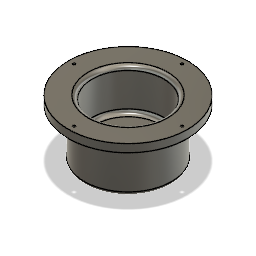
distance sensing base v1 (Autodesk Fusion 360 design; units mm, degrees)
Autodesk Fusion 360 part; units mm, degrees
note: some values were not read from the file. Set by a fixed rule: which sketch regions a step uses.
sketch "Sketch1" plane through (0, 0, 0) normal (0, 0, 1) x (1, 0, 0)
  line L0 (0, 0) -> (0, -69.4878)
  line L1 (15, -30) -> (25, -50)
  line L2 (15, -30) -> (40, -30)
  line L3 (25, -50) -> (50, -50)
  line L4 (45, -25) -> (45, 16.9)
  line L5 (55, -45) -> (55, 6.9)
  line L6 (50, 21.9) -> (75, 21.9)
  line L7 (60, 11.9) -> (75, 11.9)
  line L8 (75, 21.9) -> (75, 11.9)
  arc A0 (40, -30) -> (45, -25) centre (40, -25) ccw
  arc A1 (50, -50) -> (55, -45) centre (50, -45) ccw
  arc A2 (60, 11.9) -> (55, 6.9) centre (60, 6.9) ccw
  arc A3 (50, 21.9) -> (45, 16.9) centre (50, 16.9) ccw
  point P0 (15, -30)
  point P1 (25, -50)
  point P2 (45, -30)
  point P3 (55, -50)
  point P4 (45, 21.9)
  point P5 (55, 11.9)
  dimension "d2" = 15
  dimension "d4" = 25
  dimension "d19" = 30
  dimension "d20" = 30
  dimension "d21" = 51.9
  dimension "d22" = 61.9
  dimension "d23" = 30
  dimension "d24" = 20
  dimension "d25" = 5
  measures "d2" distance of L0 P0
  measures "d4" distance of L0 P1
  measures "d19" distance of P0 P2
  measures "d20" distance of P1 P3
  measures "d21" distance of P2 P4
  measures "d22" distance of P3 P5
  measures "d23" distance of P4 L6.end
  measures "d24" distance of P5 L7.end
  measures "d25" radius of A0
revolve "Revolve1" add sketch "Sketch1" angle 360 about axis through (0, 0, 0) along (0, -1, 0)
sketch "Sketch2" plane through (0, 0, 0) normal (0, 1, 0) x (1, 0, 0)
  circle A0 centre (-68, 0) radius 1.5
  line L0 (-68, 0) -> (0, 0)
  circle A1 centre (0, -68) radius 1.5
  circle A2 centre (68, 0) radius 1.5
  circle A3 centre (0, 68) radius 1.5
  dimension "d13" = 3
  dimension "d14" = 68
  dimension "d16" = 360
  measures "d13" diameter of A0
  measures "d14" distance of A0.centre L0.end
extrude "Extrude1" cut sketch "Sketch2" along normal mid plane 200
